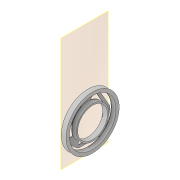
# Autodesk Inventor part: 00_Spiral_v2 v4
Saved by Autodesk Inventor 2019 (Build 230136000, 136)
## iProperties
Created: 2019-01-28
Part Number: 00_Spiral_v2 v4
Material: Stahl
Document SubType Name: Modeling
Designer: diederichbenedict
Density: 7.85 g/cm^3
Appearance: Default
Sending System: Autodesk Translation Framework v7.6.0.251
Preprocessor: ST-DEVELOPER v17.2
Title: /var/folders/4w/k4yhf14j7xsbp2jd85yk555r0000gn/T/com.autodesk.mas.fusion360/Neutron/425bdb84-621c-4cb9-a3fc-79afa15c9f79.stp
Author: benedict.diederichJXUDS
Autodesk Inventor part; units mm, degrees
note: some values were not read from the file. Chosen so that the rebuilt part matches the saved one: sketch regions of "Extrusion2".
ref_plane "YZ Plane" through (0, 0, 0) normal (1, 0, 0) x (0, 1, 0)
ref_plane "XZ Plane" through (0, 0, 0) normal (0, 1, 0) x (-1, 0, 0)
ref_plane "XY Plane" through (0, 0, 0) normal (0, 0, 1) x (1, 0, 0)
ref_plane "Work Plane2" through (0, 74.9, 24.9) normal (1, 0, 0) x (0, -1, 0)
sketch "Sketch2" plane through (0, 74.9, 24.9) normal (1, 0, 0) x (0, -1, 0)
  arc A0 (89.503, 45.1917) -> (85, 47.769) centre (74.9, 24.9) ccw construction
  line L0 (85, 47.769) -> (65, 47.769) construction
  line L1 (65, 47.769) -> (65, 47.8563) construction
  arc A1 (65, 47.8563) -> (54.6785, 39.6) centre (74.9, 24.9) ccw construction
  line L2 (52.6785, 39.6) -> (54.6785, 39.6) construction
  arc A2 (49.6785, 42.6) -> (52.6785, 39.6) centre (52.6785, 42.6) ccw construction
  line L3 (49.6785, 46.9) -> (49.6785, 42.6) construction
  arc A3 (49.6785, 46.9) -> (46.6785, 49.9) centre (46.6785, 46.9) ccw construction
  line L4 (8.3, 49.9) -> (46.6785, 49.9) construction
  line L5 (8.3, 49.9) -> (8.3, 45.9) construction
  line L6 (18.8923, 45.9) -> (8.3, 45.9) construction
  line L7 (18.8923, 45.9) -> (18.8923, 40.7294) construction
  line L8 (18.8923, 40.7294) -> (43.8923, 40.7294) construction
  line L9 (43.8923, 40.7294) -> (43.8923, 32.95) construction
  line L10 (43.8923, 32.95) -> (49.6423, 32.95) construction
  line L11 (49.6423, 32.95) -> (49.6423, 35.0971) construction
  arc A4 (50.8639, 31.775) -> (49.6423, 35.0971) centre (47.9796, 32.6) ccw construction
  arc A5 (50.8639, 31.775) -> (50.8639, 18.025) centre (74.9, 24.9) ccw construction
  arc A6 (49.6423, 14.7029) -> (50.8639, 18.025) centre (47.9796, 17.2) ccw construction
  line L12 (49.6423, 14.7029) -> (49.6423, 16.85) construction
  line L13 (49.6423, 16.85) -> (43.8923, 16.85) construction
  line L14 (43.8923, 16.85) -> (43.8923, 9.0706) construction
  line L15 (43.8923, 9.0706) -> (18.8923, 9.0706) construction
  line L16 (18.8923, 9.0706) -> (18.8923, 3.9) construction
  line L17 (18.8923, 3.9) -> (8.3, 3.9) construction
  line L18 (8.3, 3.9) -> (8.3, -0.1) construction
  line L19 (8.3, -0.1) -> (46.6785, -0.1) construction
  arc A7 (46.6785, -0.1) -> (49.6785, 2.9) centre (46.6785, 2.9) ccw construction
  line L20 (49.6785, 2.9) -> (49.6785, 7.2) construction
  arc A8 (52.6785, 10.2) -> (49.6785, 7.2) centre (52.6785, 7.2) ccw construction
  line L21 (52.6785, 10.2) -> (53.2041, 10.2) construction
  arc A9 (55.5287, 9.0964) -> (53.2041, 10.2) centre (53.2041, 7.2) ccw construction
  arc A10 (55.5287, 9.0964) -> (65, 1.9437) centre (74.9, 24.9) ccw construction
  line L22 (65, 1.9437) -> (65, 2.031) construction
  line L23 (65, 2.031) -> (85, 2.031) construction
  arc A11 (85, 2.031) -> (89.503, 4.6083) centre (74.9, 24.9) ccw construction
  line L24 (91.5, 4.6083) -> (89.503, 4.6083) construction
  line L25 (91.5, 8.3) -> (91.5, 4.6083) construction
  line L26 (91.5, 8.3) -> (98.003, 8.3) construction
  line L27 (98.003, 8.3) -> (98.003, 41.5) construction
  line L28 (98.003, 41.5) -> (91.5, 41.5) construction
  line L29 (91.5, 41.5) -> (91.5, 45.1917) construction
  line L30 (91.5, 45.1917) -> (89.503, 45.1917) construction
  circle A12 centre (26.0079, 7.4) radius 1.4 construction
  circle A13 centre (26.0079, 42.4) radius 1.4 construction
  line L31 (76.4554, 38.5617) -> (74.3635, 38.1391) projected
  arc A14 (74.3635, 38.1391) -> (67.1199, 19.4377) centre (78.6098, 25.7409) ccw projected
  line L32 (67.1199, 19.4377) -> (67.7252, 19.8946) projected
  arc A15 (76.9716, 37.9871) -> (67.7252, 19.8946) centre (78.6098, 25.7409) ccw projected
  line L33 (76.9716, 37.9871) -> (79.118, 37.9871) projected
  arc A16 (86.2186, 17.0928) -> (79.118, 37.9871) centre (74.9, 24.9) ccw projected
  line L34 (86.2186, 17.0928) -> (86.6337, 18.7451) projected
  arc A17 (86.6337, 18.7451) -> (74.0596, 34.3689) centre (73.7733, 21.2668) ccw projected
  line L35 (74.0596, 34.3689) -> (74.1525, 33.6162) projected
  arc A18 (85.1979, 16.5624) -> (74.1525, 33.6162) centre (73.7733, 21.2668) ccw projected
  line L36 (85.1979, 16.5624) -> (84.4501, 15.0076) projected
  arc A19 (62.5793, 18.7957) -> (84.4501, 15.0076) centre (74.9, 24.9) ccw projected
  line L37 (62.5793, 18.7957) -> (63.7028, 17.8158) projected
  arc A20 (63.7028, 17.8158) -> (83.5205, 20.8933) centre (72.3169, 27.6923) ccw projected
  line L38 (83.5205, 20.8933) -> (82.8222, 21.1892) projected
  arc A21 (62.5305, 20.1505) -> (82.8222, 21.1892) centre (72.3169, 27.6923) ccw projected
  line L39 (62.5305, 20.1505) -> (61.5394, 21.651) projected
  arc A22 (76.4554, 38.5617) -> (61.5394, 21.651) centre (74.9, 24.9) ccw projected
  arc A23 (75.7159, 39.8778) -> (60.1158, 27.435) centre (74.9, 24.9) ccw projected
  arc A24 (58.0807, 27.9614) -> (60.1158, 27.435) centre (59.3662, 28.7343) ccw projected
  line L40 (58.0807, 27.9614) -> (57.9635, 28.1564) projected
  arc A25 (57.9635, 28.1564) -> (55.1917, 27.586) centre (56.678, 27.3834) ccw projected
  arc A26 (55.1917, 27.586) -> (58.3649, 13.8446) centre (74.9, 24.9) ccw projected
  arc A27 (58.3649, 13.8446) -> (58.8619, 13.3792) centre (59.6119, 14.6783) ccw projected
  line L41 (58.8619, 13.3792) -> (74.6797, 4.2468) projected
  arc A28 (75.3583, 3.4049) -> (74.6797, 4.2468) centre (73.9297, 2.9478) ccw projected
  arc A29 (53.4072, 25.4575) -> (75.3583, 3.4049) centre (74.9, 24.9) ccw projected
  arc A30 (57.8704, 32.9616) -> (53.4072, 25.4575) centre (62.3367, 25.2259) ccw projected
  line L42 (57.8704, 32.9616) -> (73.8658, 42.1965) projected
  arc A31 (75.7159, 39.8778) -> (73.8658, 42.1965) centre (74.6158, 40.8975) ccw projected
  circle A32 centre (44.9, 44.9) radius 1.45 construction
  circle A33 centre (44.9, 4.9) radius 1.45 construction
  arc A34 (61.5209, 18.1177) -> (80.0967, 10.829) centre (74.9, 24.9) ccw projected
  arc A35 (80.6584, 8.8034) -> (80.0967, 10.829) centre (79.3463, 9.5302) ccw projected
  line L43 (80.6584, 8.8034) -> (80.5482, 8.6044) projected
  arc A36 (80.5482, 8.6044) -> (82.428, 6.4891) centre (81.8603, 7.8775) ccw projected
  arc A37 (82.428, 6.4891) -> (92.7418, 16.1079) centre (74.9, 24.9) ccw projected
  arc A38 (92.7418, 16.1079) -> (92.8963, 16.771) centre (91.3963, 16.771) ccw projected
  line L44 (92.8963, 16.771) -> (92.8963, 35.0358) projected
  arc A39 (93.2861, 36.0445) -> (92.8963, 35.0358) centre (94.3963, 35.0358) ccw projected
  arc A40 (96.4, 24.9) -> (93.2861, 36.0445) centre (74.9, 24.9) ccw projected
  spline S0 degree 3 poles (96.4, 24.9) (96.344, 22.8739) (95.9001, 20.9098) (94.2008, 16.5484) (92.7552, 14.2515) (89.3438, 9.943) (87.3173, 7.9149) (85.1636, 6.008) knots 0 0 0 0 0.608049 0.608049 1.404149 1.404149 2.256385 2.256385 2.256385 2.256385 projected
  arc A41 (76.4332, 6.1212) -> (85.1636, 6.008) centre (80.8994, 13.8569) ccw projected
  line L45 (76.4332, 6.1212) -> (60.4379, 15.3561) projected
  arc A42 (61.5209, 18.1177) -> (60.4379, 15.3561) centre (61.1879, 16.6551) ccw projected
  line L46 (88.5809, 40.6416) -> (88.5809, 37.9063) projected
  line L47 (88.5809, 37.9063) -> (90.098, 37.9063) projected
  arc A43 (90.3963, 35.6172) -> (90.098, 37.9063) centre (81.4639, 35.6172) ccw projected
  line L48 (90.3963, 35.6172) -> (90.3963, 17.1474) projected
  arc A44 (87.4632, 16.7045) -> (90.3963, 17.1474) centre (88.8963, 17.1474) ccw projected
  arc A45 (87.4632, 16.7045) -> (84.4875, 36.436) centre (74.9, 24.9) ccw projected
  arc A46 (85.9609, 37.9352) -> (84.4875, 36.436) centre (85.9875, 36.4355) ccw projected
  line L49 (85.9609, 37.9352) -> (86.1884, 37.9393) projected
  arc A47 (86.1884, 37.9393) -> (87.0803, 40.6249) centre (86.1617, 39.4391) ccw projected
  arc A48 (87.0803, 40.6249) -> (73.5933, 44.7475) centre (74.9, 24.9) ccw projected
  arc A49 (73.5933, 44.7475) -> (72.9418, 44.5498) centre (73.6918, 43.2508) ccw projected
  line L50 (72.9418, 44.5498) -> (57.124, 35.4174) projected
  arc A50 (56.0555, 35.2506) -> (57.124, 35.4174) centre (56.374, 36.7164) ccw projected
  arc A51 (86.1292, 43.2345) -> (56.0555, 35.2506) centre (74.9, 24.9) ccw projected
  arc A52 (87.1251, 42.5265) -> (86.1292, 43.2345) centre (81.4639, 35.6172) ccw projected
  arc A53 (88.5809, 40.6416) -> (87.1251, 42.5265) centre (83.0911, 37.9063) ccw projected
  arc A54 (84.4501, 15.0076) -> (86.2186, 17.0928) centre (74.9, 24.9) ccw
  arc A55 (79.118, 37.9871) -> (76.4554, 38.5617) centre (74.9, 24.9) ccw
  circle A56 centre (74.9, 24.9) radius 24.5087
  arc A57 (61.5394, 21.651) -> (62.5793, 18.7957) centre (69.4639, 22.9202) ccw
  point P0 (74.9, 24.9)
  constraints: 6 point on circle, 4 centre point, 1 coincident
extrude "Extrusion1" add sketch "Sketch2" along normal blind 0.45
sketch "Sketch3" plane through (0.45, 0, 0) normal (1, 0, 0) x (0, 0, -1)
  arc A0 (13.6617, -1.5554) -> (-3.249, 13.3606) centre (0, 0) ccw projected
  circle A1 centre (0, 0) radius 13.75
  circle A2 centre (0, 0) radius 15.0438
  arc A3 (-6.1043, 12.3207) -> (13.0871, -4.218) centre (0, 0) ccw projected
  arc A4 (-3.249, 13.3606) -> (-6.1043, 12.3207) centre (-1.9798, 5.4361) ccw projected
  arc A5 (13.6617, -1.5554) -> (-3.249, 13.3606) centre (0, 0) ccw projected
  arc A6 (13.0871, -4.218) -> (13.6617, -1.5554) centre (0, 0) ccw projected
  arc A7 (3.0614, 16.8193) -> (2.535, 14.7842) centre (3.8343, 15.5338) ccw projected
  line L0 (3.0614, 16.8193) -> (3.2564, 16.9365) projected
  arc A8 (3.2564, 16.9365) -> (2.686, 19.7083) centre (2.4834, 18.222) ccw projected
  arc A9 (2.686, 19.7083) -> (-11.0554, 16.5351) centre (0, 0) ccw projected
  arc A10 (-11.0554, 16.5351) -> (-11.5208, 16.0381) centre (-10.2217, 15.2881) ccw projected
  line L1 (-11.5208, 16.0381) -> (-20.6532, 0.2203) projected
  arc A11 (-21.4951, -0.4583) -> (-20.6532, 0.2203) centre (-21.9522, 0.9703) ccw projected
  arc A12 (0.5575, 21.4928) -> (-21.4951, -0.4583) centre (0, 0) ccw projected
  arc A13 (8.0616, 17.0296) -> (0.5575, 21.4928) centre (0.3259, 12.5633) ccw projected
  line L2 (8.0616, 17.0296) -> (17.2965, 1.0342) projected
  arc A14 (14.9778, -0.8159) -> (17.2965, 1.0342) centre (15.9975, 0.2842) ccw projected
  arc A15 (14.9778, -0.8159) -> (2.535, 14.7842) centre (0, 0) ccw projected
  line L3 (13.0063, -13.6809) -> (13.0063, -15.198) projected
  arc A16 (10.7172, -15.4963) -> (13.0063, -15.198) centre (10.7172, -6.5639) ccw projected
  line L4 (10.7172, -15.4963) -> (-7.7526, -15.4963) projected
  arc A17 (-8.1955, -12.5632) -> (-7.7526, -15.4963) centre (-7.7526, -13.9963) ccw projected
  arc A18 (-8.1955, -12.5632) -> (11.536, -9.5875) centre (0, 0) ccw projected
  arc A19 (13.0352, -11.0609) -> (11.536, -9.5875) centre (11.5355, -11.0875) ccw projected
  line L5 (13.0352, -11.0609) -> (13.0393, -11.2884) projected
  arc A20 (13.0393, -11.2884) -> (15.7249, -12.1803) centre (14.5391, -11.2617) ccw projected
  arc A21 (15.7249, -12.1803) -> (19.8475, 1.3067) centre (0, 0) ccw projected
  arc A22 (19.8475, 1.3067) -> (19.6498, 1.9582) centre (18.3508, 1.2082) ccw projected
  line L6 (19.6498, 1.9582) -> (10.5174, 17.776) projected
  arc A23 (10.3506, 18.8445) -> (10.5174, 17.776) centre (11.8164, 18.526) ccw projected
  arc A24 (18.3345, -11.2292) -> (10.3506, 18.8445) centre (0, 0) ccw projected
  arc A25 (17.6265, -12.2251) -> (18.3345, -11.2292) centre (10.7172, -6.5639) ccw projected
  arc A26 (15.7416, -13.6809) -> (17.6265, -12.2251) centre (13.0063, -8.1911) ccw projected
  line L7 (15.7416, -13.6809) -> (13.0063, -13.6809) projected
  arc A27 (-16.0966, -5.7584) -> (-14.071, -5.1967) centre (-15.3698, -4.4463) ccw projected
  line L8 (-16.0966, -5.7584) -> (-16.2956, -5.6482) projected
  arc A28 (-16.2956, -5.6482) -> (-18.4109, -7.528) centre (-17.0225, -6.9603) ccw projected
  arc A29 (-18.4109, -7.528) -> (-8.7921, -17.8418) centre (0, 0) ccw projected
  arc A30 (-8.7921, -17.8418) -> (-8.129, -17.9963) centre (-8.129, -16.4963) ccw projected
  line L9 (-8.129, -17.9963) -> (10.1358, -17.9963) projected
  arc A31 (11.1445, -18.3861) -> (10.1358, -17.9963) centre (10.1358, -19.4963) ccw projected
  arc A32 (0, -21.5) -> (11.1445, -18.3861) centre (0, 0) ccw projected
  arc A33 (-18.7788, -1.5332) -> (-18.892, -10.2636) centre (-11.0431, -5.9994) ccw projected
  line L10 (-18.7788, -1.5332) -> (-9.5439, 14.4621) projected
  arc A34 (-6.7823, 13.3791) -> (-9.5439, 14.4621) centre (-8.2449, 13.7121) ccw projected
  arc A35 (-6.7823, 13.3791) -> (-14.071, -5.1967) centre (0, 0) ccw projected
  circle A36 centre (0, 0) radius 24.5087 projected
  circle A37 centre (0, 0) radius 24.5
  circle A38 centre (0, 0) radius 21.5
  point P0 (0, 0)
  dimension "d4" = 49
  constraints: 4 centre point, 4 coincident, 1 concentric, 1 other
  measures "d4" diameter of A37
extrude "Extrusion2" add sketch "Sketch3" along normal blind 4 contours A1 A4 | A2 A14 A15 A7 | A7 A15 A14 A2 A19 A18 A17 A27 A35 A34 | A34 A35 A27 A2 | A2 A17 A18 A19 | A36 | A37
sketch "Sketch4" plane through (0, 0, 0) normal (-1, 0, 0) x (0, 0, 1)
  circle A0 centre (0, 0) radius 24.5087 projected
  arc A1 (-13.0871, -4.218) -> (6.1043, 12.3207) centre (0, 0) ccw projected
  arc A2 (-13.6617, -1.5554) -> (-13.0871, -4.218) centre (0, 0) ccw projected
  arc A3 (3.249, 13.3606) -> (-13.6617, -1.5554) centre (0, 0) ccw projected
  arc A4 (6.1043, 12.3207) -> (3.249, 13.3606) centre (1.9798, 5.4361) ccw projected
  arc A5 (14.071, -5.1967) -> (16.0966, -5.7584) centre (15.3698, -4.4463) ccw projected
  arc A6 (14.071, -5.1967) -> (6.7823, 13.3791) centre (0, 0) ccw projected
  arc A7 (9.5439, 14.4621) -> (6.7823, 13.3791) centre (8.2449, 13.7121) ccw projected
  line L0 (9.5439, 14.4621) -> (18.7788, -1.5332) projected
  arc A8 (18.892, -10.2636) -> (18.7788, -1.5332) centre (11.0431, -5.9994) ccw projected
  arc A9 (-11.1445, -18.3861) -> (0, -21.5) centre (0, 0) ccw projected
  arc A10 (-10.1358, -17.9963) -> (-11.1445, -18.3861) centre (-10.1358, -19.4963) ccw projected
  line L1 (-10.1358, -17.9963) -> (8.129, -17.9963) projected
  arc A11 (8.129, -17.9963) -> (8.7921, -17.8418) centre (8.129, -16.4963) ccw projected
  arc A12 (8.7921, -17.8418) -> (18.4109, -7.528) centre (0, 0) ccw projected
  arc A13 (18.4109, -7.528) -> (16.2956, -5.6482) centre (17.0225, -6.9603) ccw projected
  line L2 (16.2956, -5.6482) -> (16.0966, -5.7584) projected
  line L3 (-13.0063, -15.198) -> (-13.0063, -13.6809) projected
  line L4 (-13.0063, -13.6809) -> (-15.7416, -13.6809) projected
  arc A14 (-17.6265, -12.2251) -> (-15.7416, -13.6809) centre (-13.0063, -8.1911) ccw projected
  arc A15 (-18.3345, -11.2292) -> (-17.6265, -12.2251) centre (-10.7172, -6.5639) ccw projected
  arc A16 (-10.3506, 18.8445) -> (-18.3345, -11.2292) centre (0, 0) ccw projected
  arc A17 (-10.5174, 17.776) -> (-10.3506, 18.8445) centre (-11.8164, 18.526) ccw projected
  line L5 (-10.5174, 17.776) -> (-19.6498, 1.9582) projected
  arc A18 (-19.6498, 1.9582) -> (-19.8475, 1.3067) centre (-18.3508, 1.2082) ccw projected
  arc A19 (-19.8475, 1.3067) -> (-15.7249, -12.1803) centre (0, 0) ccw projected
  arc A20 (-15.7249, -12.1803) -> (-13.0393, -11.2884) centre (-14.5391, -11.2617) ccw projected
  line L6 (-13.0393, -11.2884) -> (-13.0352, -11.0609) projected
  arc A21 (-11.536, -9.5875) -> (-13.0352, -11.0609) centre (-11.5355, -11.0875) ccw projected
  arc A22 (-11.536, -9.5875) -> (8.1955, -12.5632) centre (0, 0) ccw projected
  arc A23 (7.7526, -15.4963) -> (8.1955, -12.5632) centre (7.7526, -13.9963) ccw projected
  line L7 (7.7526, -15.4963) -> (-10.7172, -15.4963) projected
  arc A24 (-13.0063, -15.198) -> (-10.7172, -15.4963) centre (-10.7172, -6.5639) ccw projected
  arc A25 (-2.535, 14.7842) -> (-3.0614, 16.8193) centre (-3.8343, 15.5338) ccw projected
  arc A26 (-2.535, 14.7842) -> (-14.9778, -0.8159) centre (0, 0) ccw projected
  arc A27 (-17.2965, 1.0342) -> (-14.9778, -0.8159) centre (-15.9975, 0.2842) ccw projected
  line L8 (-17.2965, 1.0342) -> (-8.0616, 17.0296) projected
  arc A28 (-0.5575, 21.4928) -> (-8.0616, 17.0296) centre (-0.3259, 12.5633) ccw projected
  arc A29 (21.4951, -0.4583) -> (-0.5575, 21.4928) centre (0, 0) ccw projected
  arc A30 (20.6532, 0.2203) -> (21.4951, -0.4583) centre (21.9522, 0.9703) ccw projected
  line L9 (20.6532, 0.2203) -> (11.5208, 16.0381) projected
  arc A31 (11.5208, 16.0381) -> (11.0554, 16.5351) centre (10.2217, 15.2881) ccw projected
  arc A32 (11.0554, 16.5351) -> (-2.686, 19.7083) centre (0, 0) ccw projected
  arc A33 (-2.686, 19.7083) -> (-3.2564, 16.9365) centre (-2.4834, 18.222) ccw projected
  line L10 (-3.2564, 16.9365) -> (-3.0614, 16.8193) projected
  arc A34 (-13.0063, -15.198) -> (-10.7172, -15.4963) centre (-10.7172, -6.5639) ccw projected
  arc A35 (-10.7172, -15.4963) -> (7.7526, -15.6136) centre (-0.3886, 156.7571) ccw
  arc A36 (18.892, -10.2636) -> (18.7788, -1.5332) centre (11.0431, -5.9994) ccw projected
  line L11 (18.7788, -1.5332) -> (9.5439, 14.4621) projected
  arc A37 (18.7788, -1.5332) -> (9.5439, 14.4621) centre (-49.6016, -30.3491) ccw
  arc A38 (-0.5575, 21.4928) -> (-8.0616, 17.0296) centre (-0.3259, 12.5633) ccw projected
  arc A39 (-8.0616, 17.0296) -> (-17.2965, 1.0342) centre (51.644, -28.105) ccw
  line L12 (-13.0063, -13.6809) -> (-15.7416, -13.6809) projected
  arc A40 (-15.7416, -13.6809) -> (-13.0063, -15.198) centre (-12.0947, -10.33) ccw
  arc A41 (0, -21.5) -> (18.892, -10.2636) centre (0, 0) ccw projected
  spline S0 degree 3 poles (0, -21.5) (2.0261, -21.444) (3.9902, -21.0001) (8.3516, -19.3008) (10.6485, -17.8552) (14.957, -14.4438) (16.9851, -12.4173) (18.892, -10.2636) knots 0 0 0 0 0.269479 0.269479 0.6223 0.6223 1 1 1 1 projected
  point P0 (0, 0)
  constraints: 10 point on circle, 4 centre point, 1 point on line, 2 other
extrude "Extrusion3" cut sketch "Sketch4" against normal through all contours A41 S0 | A40 L4 L3
body "Solid2"
